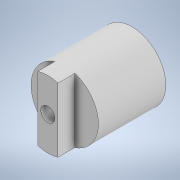
# Autodesk Inventor part: Ender 5 Foot Spacer
Saved by Autodesk Inventor 2021 (Build 250183000, 183)
## iProperties
Created: 2021-03-20
Part Number: Ender 5 Foot Spacer
Material: Generic
Document SubType Name: Modeling
Designer: alexr
Density: 1 g/cm^3
Appearance: Default
Author: alexr
Autodesk Inventor part; units mm, degrees
ref_plane "YZ Plane" through (0, 0, 0) normal (1, 0, 0) x (0, 1, 0)
ref_plane "XZ Plane" through (0, 0, 0) normal (0, 1, 0) x (-1, 0, 0)
ref_plane "XY Plane" through (0, 0, 0) normal (0, 0, 1) x (1, 0, 0)
sketch "Sketch1" plane through (0, 0, 0) normal (0, 0, 1) x (1, 0, 0)
  circle A0 centre (0, 0) radius 10
  dimension "d0" = 20
  constraints: 1 centre point, 1 coincident
  measures "d0" diameter of A0
extrude "Extrusion1" add sketch "Sketch1" along normal blind 20
sketch "Sketch2" plane through (0, 0, 20) normal (0, 0, 1) x (1, 0, 0)
  circle A0 centre (0, 0) radius 10 projected
  line L0 (0, 10) -> (0, -10) construction
  line L1 (3, 9.5394) -> (3, -9.5394)
  line L2 (-3, 9.5394) -> (-3, -9.5394)
  arc A1 (-3, -9.5394) -> (3, -9.5394) centre (0, 0) ccw
  arc A2 (3, 9.5394) -> (-3, 9.5394) centre (0, 0) ccw
  dimension "d3" = 3
  dimension "d4" = 3
  constraints: 6 end point, 6 point on circle, 2 centre point, 2 parallel, 8 other
  measures "d3" distance between parallel lines of L0 L1
  measures "d4" distance between parallel lines of L0 L2
extrude "Extrusion2" add sketch "Sketch2" along normal blind 5 contours L1 A0 L2
hole "Hole1" at (0, 0, 0) direction (0, 0, 1) diameter 4.2 end through all
body "Solid1"
